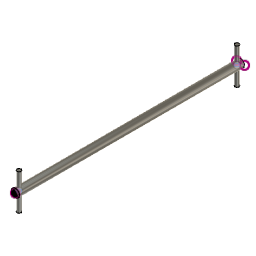
Front Dogbone (Autodesk Fusion 360 design; units mm, degrees)
Autodesk Fusion 360 part; units mm, degrees
sketch "Sketch1" plane through (0, 0, 0) normal (0, 1, 0) x (1, 0, 0)
  circle A0 centre (0, 0) radius 2
  dimension "d5" = 4
  constraint coincident A0.centre origin
  measures "d5" diameter of A0
extrude "Extrude1" add sketch "Sketch1" along normal blind 113 makes body 1
sketch "Sketch2" plane through (0, 0, 0) normal (0, 0, 1) x (1, 0, 0)
  circle A0 centre (0, 1.8) radius 1
  circle A1 centre (0, 111.2) radius 1
  line L0 (2, 113) -> (-2, 113)
  dimension "d9" = 2
  dimension "d10" = 2
  dimension "d15" = 1.8
  dimension "d16" = 1.8
  measures "d9" diameter of A0
  measures "d10" diameter of A1
  measures "d15" distance of A0.centre origin
  measures "d16" distance of A1.centre L0
extrude "Extrude2" add sketch "Sketch2" along normal mid plane 18 separate body contours A1 makes body 2
extrude "Extrude3" add sketch "Sketch2" along normal mid plane 18 separate body contours A0 makes body 3
equation "length = 113 mm"
equation "radius = 2 mm"
equation "cup_little_bone_radius = 1 mm"
equation "cup_little_bone_length = 18 mm"
equation "d5 = radius * 2"
equation "edge_cup_little_bone_distance = 1.8 mm"
equation "d7 = length"
equation "d9 = cup_little_bone_radius * 2"
equation "d10 = cup_little_bone_radius * 2"
equation "d11 = cup_little_bone_length / 2"
equation "d13 = cup_little_bone_length / 2"
equation "d15 = edge_cup_little_bone_distance"
equation "d16 = edge_cup_little_bone_distance"
